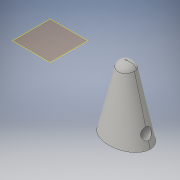
# Autodesk Inventor part: landing
Saved by Autodesk Inventor 2016 (Build 200138000, 138)
## iProperties
Created: 2015-08-30
Part Number: landing
Material: Generic
Document SubType Name: Modeling
Designer: adam
Density: 1 g/cm^3
Appearance: Default
Author: adam
Autodesk Inventor part; units mm, degrees
ref_plane "YZ Plane" through (0, 0, 0) normal (1, 0, 0) x (0, 1, 0)
ref_plane "XZ Plane" through (0, 0, 0) normal (0, 1, 0) x (-1, 0, 0)
ref_plane "XY Plane" through (0, 0, 0) normal (0, 0, 1) x (1, 0, 0)
sketch "Sketch1" plane through (0, 0, 0) normal (0, 1, 0) x (-1, 0, 0)
  ellipse E0 centre (0, 0) end of major axis (14, 0) minor radius 10
  dimension "d0" = 10
  dimension "d1" = 14
  constraints: 1 coincident, 2 other
ref_plane "Work Plane4" through (0, 38, 0) normal (0, 1, 0) x (1, 0, 0)
sketch "Sketch8" plane through (0, 38, 0) normal (0, 1, 0) x (1, 0, 0)
  circle A0 centre (0, 0) radius 4
  dimension "d13" = 8
  constraints: 1 centre point, 1 coincident
  measures "d13" diameter of A0
loft "Loft2" add profiles "Sketch1", "Sketch8"
fillet "Fillet3" radius 4.29 2 edges at (0, 38, 4) (0, 38, -4)
sketch "Sketch9" plane through (0, 0, 0) normal (1, 0, 0) x (0, 1, 0)
  line L0 (0, 0) -> (34.8018, 0) projected
  circle A0 centre (7, 0) radius 3
  dimension "d20" = 6
  dimension "d21" = 7
  constraints: 1 centre point, 1 point on line
  measures "d20" diameter of A0
  measures "d21" distance of L0.start A0.centre
extrude "Extrusion2" cut sketch "Sketch9" along normal through all both and the other way through all
body "Solid3"
